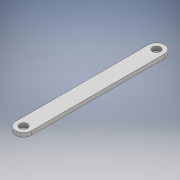
# Autodesk Inventor part: 連桿4
Saved by Autodesk Inventor 2017 (Build 210142000, 142)
## iProperties
Part Number: 連桿4
Material: 一般
Document SubType Name: Modeling
Designer: user
Density: 1 g/cm^3
Appearance: 預設
Author: user
Autodesk Inventor part; units mm, degrees
ref_plane "YZ Plane" through (0, 0, 0) normal (1, 0, 0) x (0, 1, 0)
ref_plane "XZ Plane" through (0, 0, 0) normal (0, 1, 0) x (-1, 0, 0)
ref_plane "XY Plane" through (0, 0, 0) normal (0, 0, 1) x (1, 0, 0)
sketch "草圖1" plane through (0, 0, 0) normal (0, 0, 1) x (1, 0, 0)
  line L0 (0, -16.62) -> (0, 16.62) construction
  line L1 (2, -16.62) -> (2, 16.62)
  line L2 (-2, 16.62) -> (-2, -16.62)
  arc A0 (-2, -16.62) -> (2, -16.62) centre (0, -16.62) ccw
  arc A1 (2, 16.62) -> (-2, 16.62) centre (0, 16.62) ccw
  point P0 (0, 0)
  dimension "d0" = 33.24
  dimension "d1" = 4
  constraints: 8 end point, 4 point on circle, 4 tangent, 2 centre point, 1 midpoint, 1 parallel, 1 vertical
  measures "d0" distance of L0.start L0.end
  measures "d1" distance between parallel lines of L1 L2
extrude "擠出1" add sketch "草圖1" along normal blind 1
sketch "草圖2" plane through (0, 0, 1) normal (0, 0, 1) x (1, 0, 0)
  arc A0 (2, 16.62) -> (-2, 16.62) centre (0, 16.62) ccw projected
  circle A1 centre (0, 16.62) radius 0.75
  arc A2 (-2, -16.62) -> (2, -16.62) centre (0, -16.62) ccw projected
  circle A3 centre (0, -16.62) radius 0.75
  point P0 (0, 0)
  dimension "d4" = 1.5
  dimension "d5" = 1.5
  constraints: 2 centre point, 2 coincident
  measures "d4" diameter of A1
  measures "d5" diameter of A3
extrude "擠出2" add sketch "草圖2" along normal blind 1
hole "孔1" at (0, -16.62, 1) at (0, 16.62, 1) direction (0, 0, -1) diameter 2 end through all
hole "孔2" at (0, -16.62, 1) at (0, 16.62, 1) direction (0, 0, 1) diameter 2 end through all
